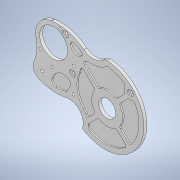
# Autodesk Inventor part: 足内フレーム
Saved by Autodesk Inventor 2022.2 (Build 262287010, 287A)
## iProperties
Created: 2022-01-10
Part Number: 足内フレーム
Material: Aluminum 2014-T4
Document SubType Name: Modeling
Designer: acps
Density: 2.8 g/cm^3
Appearance: Satin
Author: acps
Autodesk Inventor part; units mm, degrees
ref_plane "YZ Plane" through (0, 0, 0) normal (1, 0, 0) x (0, 1, 0)
ref_plane "XZ Plane" through (0, 0, 0) normal (0, 1, 0) x (-1, 0, 0)
ref_plane "XY Plane" through (0, 0, 0) normal (0, 0, 1) x (1, 0, 0)
sketch "Sketch2" plane through (0, 0, 0) normal (0, 0, 1) x (1, 0, 0)
  circle A0 centre (46.4683, 30) radius 14
  circle A1 centre (66.4734, 20) radius 20.5 construction
  circle A2 centre (100, 0) radius 30 construction
  circle A3 centre (123.045, 25) radius 1.25
  circle A4 centre (100, 0) radius 3 construction
  circle A5 centre (35, 0) radius 6.025 construction
  circle A6 centre (35, 0) radius 9
  arc A7 (26.7096, 3.5028) -> (28.866, 26.2368) centre (-8.2942, 18.2924) ccw
  arc A8 (44, 47.83) -> (28.866, 26.2368) centre (46.4683, 30) ccw
  arc A9 (110.6259, 39.2116) -> (45.1112, 47.9488) centre (57.174, -111.5959) ccw construction
  arc A10 (91.0837, -36) -> (110.6259, 39.2116) centre (97.597, 2.4523) ccw
  arc A11 (28.683, 27.2278) -> (91.0837, -36) centre (103.7763, 38.9326) ccw construction
  circle A12 centre (58.3063, 43.4) radius 1.5
  arc A13 (44.5539, 47.9057) -> (44, 47.83) centre (65.9403, -110.6586) ccw
  arc A14 (76.7854, 39.1678) -> (44.5539, 47.9057) centre (50.3015, 5.2915) ccw
  arc A15 (76.7854, 39.1678) -> (96.2775, 40.0369) centre (86.0239, 50.9851) ccw
  arc A16 (100.004, 41.3779) -> (96.2775, 40.0369) centre (99.6954, 36.3875) ccw
  arc A17 (91.0837, -36) -> (100.004, 41.3779) centre (97.597, 2.4523) ccw
  arc A18 (75.52, -28.3291) -> (58.8706, -11.0424) centre (62.0019, -24.6877) ccw
  arc A19 (31.2271, -8.171) -> (58.8706, -11.0424) centre (49.2531, 30.8683) ccw
  arc A20 (75.52, -28.3291) -> (76.4189, -30.5623) centre (77.4512, -28.8493) ccw
  arc A21 (76.4189, -30.5623) -> (91.0837, -36) centre (98.098, 5.4101) ccw
  circle A22 centre (58.3063, 43.4) radius 1.5
  circle A23 centre (123.045, 25) radius 1.25
  circle A24 centre (100, 0) radius 3 construction
  circle A25 centre (100, 0) radius 8.525
  circle A26 centre (65.359, 13) radius 1.25
  arc A27 (131.5793, 3.5511) -> (107.9544, 34.8363) centre (97.597, 2.4523) ccw construction
  circle A28 centre (66.4734, 20) radius 1.5
  circle A29 centre (66.299, -4.4994) radius 4 construction
  circle A30 centre (66.299, -4.4994) radius 1.5
  circle A31 centre (66.299, -4.4994) radius 3 construction
  circle A32 centre (53.0056, 45.2) radius 1.25
  arc A33 (59.6568, 44.1821) -> (46.2779, 45.0886) centre (50.3015, 5.2915) ccw construction
  circle A34 centre (45.1, 8.5) radius 1.25
  circle A35 centre (33, 18) radius 1.25
  arc A36 (31.0568, 25.3067) -> (30.8433, 25.9979) centre (-68.6067, -5.1096) ccw construction
  line L0 (51.7556, 0) -> (32.0278, 0) construction
  circle A37 centre (35, 0) radius 1.5
  point P0 (0, 0)
  point P1 (0, 0)
  point P2 (86.6921, 36)
  point P3 (61.5525, 46.7935)
  point P4 (110.6259, 39.2116)
  dimension "d0" = 12.05
  dimension "d1" = 18
  dimension "d4" = 4
  dimension "d6" = 15
  dimension "d7" = 14
  dimension "d8" = 2
  dimension "d9" = 43
  dimension "d10" = 5
  dimension "d11" = 43
  dimension "d12" = 36
  dimension "d13" = 44
  dimension "d14" = 42
  dimension "d15" = 74
  dimension "d16" = 118
  dimension "d18" = 110.6259
  dimension "d21" = 17.05
  dimension "d22" = 2.5
  dimension "d23" = 37
  dimension "d24" = 13
  dimension "d26" = 3
  dimension "d27" = 2.5
  dimension "d28" = 25
  dimension "d29" = 5
  dimension "d35" = 3
  dimension "d36" = 8
  dimension "d37" = 3
  dimension "d38" = 6
  dimension "d39" = 2.5
  dimension "d40" = 3
  dimension "d42" = 45.2
  dimension "d43" = 2.5
  dimension "d44" = 8.5
  dimension "d45" = 45.1
  dimension "d46" = 2.5
  dimension "d50" = 65.359
  dimension "d51" = 35
  dimension "d52" = 38
  dimension "d53" = 18
  dimension "d54" = 33
  dimension "d116" = 3
  constraints: 41 point on circle, 37 centre point, 16 tangent, 9 coincident, 6 concentric, 2 end point, 2 horizontal, 1 point on line, 14 other
  measures "d0" diameter of A5
  measures "d1" diameter of A6
  measures "d4" radial gap between concentric circles of A8 A0
  measures "d6" radius of A15
  measures "d7" radius of A18
  measures "d8" radius of A20
  measures "d9" radius of A19
  measures "d10" radius of A16
  measures "d11" radius of A14
  measures "d12" vertical distance of point (0, 0) point (86.692, 36)
  measures "d13" horizontal distance of point (0, 0) A8.start
  measures "d14" radius of A21
  measures "d18" horizontal distance of point (0, 0) A10.end
  measures "d21" diameter of A25
  measures "d22" diameter of A26
  measures "d23" distance of A2.centre A26.centre
  measures "d24" vertical distance of point (0, 0) A26.centre
  measures "d26" diameter of A12
  measures "d27" diameter of A3
  measures "d28" vertical distance of point (0, 0) A3.centre
  measures "d29" radial gap between concentric circles of A10 A27
  measures "d35" diameter of A28
  measures "d36" diameter of A29
  measures "d37" diameter of A30
  measures "d38" diameter of A31
  measures "d39" diameter of A32
  measures "d40" radial gap between concentric circles of A14 A33
  measures "d42" vertical distance of point (0, 0) A32.centre
  measures "d43" diameter of A34
  measures "d44" vertical distance of point (0, 0) A34.centre
  measures "d45" horizontal distance of point (0, 0) A34.centre
  measures "d46" diameter of A35
  measures "d50" horizontal distance of point (0, 0) A26.centre
  measures "d51" distance of A6.centre point (0, 0)
  measures "d52" radius of A7
  measures "d53" vertical distance of point (0, 0) A35.centre
  measures "d54" horizontal distance of point (0, 0) A35.centre
  measures "d116" diameter of A37
extrude "Extrusion1" add sketch "Sketch2" against normal blind 3
sketch "Sketch3" plane through (0, 0, 0) normal (0, 0, 1) x (1, 0, 0)
  circle A0 centre (58.3063, 43.4) radius 3
  circle A1 centre (65.359, 13) radius 3
  circle A2 centre (123.045, 25) radius 1.25 projected
  circle A3 centre (123.045, 25) radius 3
  point P0 (0, 0)
  dimension "d30" = 6
  dimension "d31" = 6
  dimension "d32" = 6
  constraints: 3 centre point, 3 coincident
  measures "d30" diameter of A0
  measures "d31" diameter of A1
  measures "d32" diameter of A3
extrude "Extrusion2" cut sketch "Sketch3" against normal blind 1 contours A0 | A1 | A2 | A3
sketch "Sketch4" plane through (0, 0, 0) normal (0, 0, 1) x (1, 0, 0)
  arc A0 (83.9638, 31.0915) -> (98.805, 35.6018) centre (86.0239, 50.9851) ccw
  arc A1 (76.7854, 39.1678) -> (96.2775, 40.0369) centre (86.0239, 50.9851) ccw projected
  circle A2 centre (66.4734, 20) radius 1.5 projected
  arc A3 (91.0837, -36) -> (100.004, 41.3779) centre (97.597, 2.4523) ccw projected
  circle A4 centre (100, 0) radius 8.525 projected
  arc A5 (72.3356, 17.192) -> (72.9578, 20.4509) centre (66.4734, 20) ccw
  circle A6 centre (46.4683, 30) radius 14 projected
  arc A7 (101.0246, 36.2791) -> (98.805, 35.6018) centre (100.7221, 33.2943) ccw
  arc A8 (115.5935, 31.2989) -> (101.0246, 36.2791) centre (97.597, 2.4523) ccw
  arc A9 (117.3038, 26.7431) -> (124.0841, 19.0907) centre (123.045, 25) ccw
  circle A10 centre (123.045, 25) radius 3 projected
  arc A11 (128.4007, 16.8443) -> (124.0841, 19.0907) centre (124.7768, 15.1511) ccw
  arc A12 (83.3223, -28.406) -> (128.4007, 16.8443) centre (97.597, 2.4523) ccw
  arc A13 (81.0017, -24.7603) -> (83.3223, -28.406) centre (85.0017, -24.7756) ccw
  arc A14 (81.0017, -24.7603) -> (76.328, -12.2073) centre (62.0019, -24.6877) ccw
  arc A15 (75.52, -28.3291) -> (58.8706, -11.0424) centre (62.0019, -24.6877) ccw projected
  circle A16 centre (66.299, -4.4994) radius 1.5 projected
  circle A17 centre (100, 0) radius 15.525
  arc A18 (48.6036, -7.1262) -> (57.9971, -6.112) centre (49.2531, 30.8683) ccw
  arc A19 (44.8283, -2.0195) -> (48.6036, -7.1262) centre (48.672, -3.1268) ccw
  arc A20 (31.2271, -8.171) -> (58.8706, -11.0424) centre (49.2531, 30.8683) ccw projected
  arc A21 (72.3356, 17.192) -> (76.328, -12.2073) centre (96.6862, 5.5281) ccw
  arc A22 (48.6524, 4.6231) -> (44.8283, -2.0195) centre (60.2031, -6.4485) ccw
  arc A23 (62.2417, 5.4118) -> (48.6524, 4.6231) centre (55.8716, -2.2967) ccw
  arc A24 (62.4749, -0.5464) -> (62.2417, 5.4118) centre (59.6936, 2.3284) ccw
  arc A25 (62.4749, -0.5464) -> (60.9598, -3.1794) centre (66.299, -4.4994) ccw
  arc A26 (54.145, 12.6119) -> (43.432, 4.4478) centre (60.2031, -6.4485) ccw construction
  circle A27 centre (45.1, 8.5) radius 1.25 projected
  arc A28 (67.6549, 6.9852) -> (54.9349, 12.674) centre (55.8716, -2.2967) ccw construction
  circle A29 centre (65.359, 13) radius 3 projected
  arc A30 (57.9971, -6.112) -> (60.9598, -3.1794) centre (57.0767, -2.2194) ccw
  arc A31 (43.9376, 3.3219) -> (41.8928, -7.3744) centre (48.672, -3.1268) ccw construction
  arc A32 (83.9638, 31.0915) -> (72.9578, 20.4509) centre (82.9337, 21.1447) ccw
  arc A33 (117.3038, 26.7431) -> (115.5935, 31.2989) centre (113.4763, 27.9051) ccw
  line L0 (122.5344, -20.6589) -> (111.8754, -10)
  line L1 (119.6469, -23.4283) -> (108.9231, -12.7045)
  line L2 (117.9886, 21.77) -> (108.9231, 12.7045)
  line L3 (121.1745, 19.299) -> (111.8754, 10)
  line L4 (0, 0) -> (194.5551, 0) construction
  line L5 (91.0769, 12.7045) -> (75.7157, 28.0657)
  line L6 (88.1246, 10) -> (73.5429, 24.5817)
  line L7 (88.1246, -10) -> (79.8771, -18.2475)
  line L8 (91.0769, -12.7045) -> (80.9144, -22.867)
  arc A34 (67.721, 40.1851) -> (63.3889, 37.7183) centre (66.381, 37.5009) ccw
  arc A35 (74.5126, 35.8664) -> (67.721, 40.1851) centre (50.3015, 5.2915) ccw
  arc A36 (74.7817, 32.9878) -> (74.5126, 35.8664) centre (73.271, 34.2984) ccw
  arc A37 (63.3889, 37.7183) -> (74.7817, 32.9878) centre (69.8718, 37.2473) ccw
  arc A38 (76.7854, 39.1678) -> (44.5539, 47.9057) centre (50.3015, 5.2915) ccw projected
  arc A39 (59.4664, 38.6529) -> (65.1004, 27.8941) centre (69.8718, 37.2473) ccw construction
  arc A40 (66.3457, 44.5008) -> (59.4046, 38.0749) centre (66.381, 37.5009) ccw construction
  circle A41 centre (58.3063, 43.4) radius 3 projected
  point P0 (85.9957, -17.7858)
  dimension "d56" = 5
  dimension "d64" = 5
  dimension "d65" = 3
  dimension "d66" = 3
  dimension "d67" = 5
  dimension "d68" = 4
  dimension "d69" = 5
  dimension "d72" = 4
  dimension "d73" = 7
  dimension "d75" = 5
  dimension "d76" = 4
  dimension "d79" = 5
  dimension "d82" = 27
  dimension "d83" = 4
  dimension "d84" = 5
  dimension "d85" = 4
  dimension "d86" = 4
  dimension "d87" = 4
  dimension "d88" = 16
  dimension "d89" = 10
  dimension "d90" = 4
  dimension "d91" = 10
  dimension "d92" = 4
  dimension "d94" = 4
  dimension "d95" = 4
  dimension "d96" = 10
  dimension "d97" = 45
  dimension "d99" = 10
  dimension "d100" = 45
  dimension "d101" = 135
  dimension "d102" = 10
  dimension "d103" = 4
  dimension "d104" = 45
  dimension "d105" = 4
  dimension "d106" = 10
  dimension "d109" = 4
  dimension "d110" = 4
  dimension "d111" = 4
  dimension "d112" = 2
  dimension "d113" = 6.5
  dimension "d114" = 3
  constraints: 64 point on circle, 28 centre point, 27 tangent, 18 end point, 14 concentric, 4 parallel, 1 coincident, 1 horizontal, 1 midpoint, 10 other
  measures "d56" radial gap between concentric circles of A1 A0
  measures "d64" radial gap between concentric circles of A3 A8
  measures "d65" radius of A7
  measures "d66" radial gap between concentric circles of A9 A10
  measures "d67" radial gap between concentric circles of A12 A3
  measures "d68" radius of A11
  measures "d69" radial gap between concentric circles of A15 A14
  measures "d72" radius of A13
  measures "d75" radial gap between concentric circles of A20 A18
  measures "d76" radius of A19
  measures "d79" radial gap between concentric circles of A2 A5
  measures "d82" radius of A21
  measures "d83" radial gap between concentric circles of A22 A26
  measures "d84" radial gap between concentric circles of A23 A28
  measures "d85" radius of A24
  measures "d86" radial gap between concentric circles of A16 A25
  measures "d87" radius of A30
  measures "d88" radius of A22
  measures "d89" radius of A23
  measures "d90" radial gap between concentric circles of A31 A19
  measures "d91" radius of A32
  measures "d92" radius of A33
  measures "d94" distance between parallel lines of L0 L1
  measures "d95" distance between parallel lines of L2 L3
  measures "d96" vertical distance of L4.start L3.end
  measures "d97" angle of L4 L0
  measures "d99" vertical distance of L4.start L0.end
  measures "d100" angle of L4 L3
  measures "d101" angle of L4 L6
  measures "d102" vertical distance of L4.start L6.start
  measures "d103" distance between parallel lines of L6 L5
  measures "d104" angle of L4 L7
  measures "d105" distance from line of point (85.996, -17.786) L7
  measures "d106" vertical distance of L4.start L7.start
  measures "d109" radial gap between concentric circles of A34 A40
  measures "d110" radial gap between concentric circles of A38 A35
  measures "d111" radial gap between concentric circles of A39 A37
  measures "d112" radius of A36
  measures "d113" radius of A37
  measures "d114" radius of A34
extrude "Extrusion3" cut sketch "Sketch4" against normal blind 1.3 contours A0 A7 A8 A33 A9 L2 A17 L5 A32 | L6 A17 L7 A14 A21 A5 A32 | L3 A9 A11 A12 L0 A17 | A17 L1 A12 A13 A14 L8 | A19 A22 A23 A24 A25 A30 A18 | A35 A36 A37 A34
fillet "Fillet1" radius 2 16 edges at (111.8754, 10, -0.65) (111.8754, -10, -0.65) (122.5344, -20.6589, -0.65) (108.9231, -12.7045, -0.65) (119.6469, -23.4283, -0.65) (91.0769, -12.7045, -0.65) (88.1246, -10, -0.65) (88.1246, 10, -0.65) (73.5429, 24.5817, -0.65) (79.8771, -18.2475, -0.65) (91.0769, 12.7045, -0.65) (75.7157, 28.0657, -0.65) (108.9231, 12.7045, -0.65) (117.9886, 21.77, -0.65) (80.9144, -22.867, -0.65) (121.1745, 19.299, -0.65)
sketch "export" plane through (0, 0, 0) normal (0, 0, 1) x (1, 0, 0)
  line L0 (113.1045, 11.2291) -> (120.3869, 18.5115) projected
  arc A0 (122.1121, 19.073) -> (120.3869, 18.5115) centre (121.8011, 17.0973) ccw projected
  arc A1 (122.1121, 19.073) -> (124.0841, 19.0907) centre (123.045, 25) ccw projected
  arc A2 (128.4007, 16.8443) -> (124.0841, 19.0907) centre (124.7768, 15.1511) ccw projected
  arc A3 (123.9839, -18.9891) -> (128.4007, 16.8443) centre (97.597, 2.4523) ccw projected
  arc A4 (121.0175, -19.1421) -> (123.9839, -18.9891) centre (122.4317, -17.7279) ccw projected
  line L1 (121.0175, -19.1421) -> (113.1045, -11.2291) projected
  arc A5 (112.8618, -8.6948) -> (113.1045, -11.2291) centre (114.5187, -9.8149) ccw projected
  arc A6 (112.8618, -8.6948) -> (112.8618, 8.6948) centre (100, 0) ccw projected
  arc A7 (113.1045, 11.2291) -> (112.8618, 8.6948) centre (114.5187, 9.8149) ccw projected
  arc A8 (48.6524, 4.6231) -> (44.8283, -2.0195) centre (60.2031, -6.4485) ccw projected
  arc A9 (62.2417, 5.4118) -> (48.6524, 4.6231) centre (55.8716, -2.2967) ccw projected
  arc A10 (62.4749, -0.5464) -> (62.2417, 5.4118) centre (59.6936, 2.3284) ccw projected
  arc A11 (62.4749, -0.5464) -> (60.9598, -3.1794) centre (66.299, -4.4994) ccw projected
  arc A12 (57.9971, -6.112) -> (60.9598, -3.1794) centre (57.0767, -2.2194) ccw projected
  arc A13 (48.6036, -7.1262) -> (57.9971, -6.112) centre (49.2531, 30.8683) ccw projected
  arc A14 (44.8283, -2.0195) -> (48.6036, -7.1262) centre (48.672, -3.1268) ccw projected
  line L2 (89.9475, 13.8339) -> (77.2718, 26.5097) projected
  arc A15 (77.6241, 29.6187) -> (77.2718, 26.5097) centre (78.686, 27.9239) ccw projected
  arc A16 (83.9638, 31.0915) -> (77.6241, 29.6187) centre (82.9337, 21.1447) ccw projected
  arc A17 (83.9638, 31.0915) -> (98.805, 35.6018) centre (86.0239, 50.9851) ccw projected
  arc A18 (101.0246, 36.2791) -> (98.805, 35.6018) centre (100.7221, 33.2943) ccw projected
  arc A19 (115.5935, 31.2989) -> (101.0246, 36.2791) centre (97.597, 2.4523) ccw projected
  arc A20 (117.3038, 26.7431) -> (115.5935, 31.2989) centre (113.4763, 27.9051) ccw projected
  arc A21 (117.3038, 26.7431) -> (117.4325, 22.8787) centre (123.045, 25) ccw projected
  arc A22 (116.9759, 20.7573) -> (117.4325, 22.8787) centre (115.5617, 22.1715) ccw projected
  line L3 (116.9759, 20.7573) -> (110.0525, 13.8339) projected
  arc A23 (107.6525, 13.508) -> (110.0525, 13.8339) centre (108.6383, 15.2481) ccw projected
  arc A24 (107.6525, 13.508) -> (92.3475, 13.508) centre (100, 0) ccw projected
  arc A25 (89.9475, 13.8339) -> (92.3475, 13.508) centre (91.3617, 15.2481) ccw projected
  line L4 (110.0525, -13.8339) -> (118.0628, -21.8442) projected
  arc A26 (117.8393, -24.8653) -> (118.0628, -21.8442) centre (116.6485, -23.2584) ccw projected
  arc A27 (83.3223, -28.406) -> (117.8393, -24.8653) centre (97.597, 2.4523) ccw projected
  arc A28 (81.0017, -24.7603) -> (83.3223, -28.406) centre (85.0017, -24.7756) ccw projected
  arc A29 (81.0017, -24.7603) -> (80.978, -23.7347) centre (62.0019, -24.6877) ccw projected
  arc A30 (81.5612, -22.2202) -> (80.978, -23.7347) centre (82.9754, -23.6344) ccw projected
  line L5 (81.5612, -22.2202) -> (89.9475, -13.8339) projected
  arc A31 (92.3475, -13.508) -> (89.9475, -13.8339) centre (91.3617, -15.2481) ccw projected
  arc A32 (92.3475, -13.508) -> (107.6525, -13.508) centre (100, 0) ccw projected
  arc A33 (110.0525, -13.8339) -> (107.6525, -13.508) centre (108.6383, -15.2481) ccw projected
  line L6 (86.8955, -11.2291) -> (81.9314, -16.1932) projected
  arc A34 (78.7538, -15.7227) -> (81.9314, -16.1932) centre (80.5172, -14.779) ccw projected
  arc A35 (78.7538, -15.7227) -> (76.328, -12.2073) centre (62.0019, -24.6877) ccw projected
  arc A36 (72.3356, 17.192) -> (76.328, -12.2073) centre (96.6862, 5.5281) ccw projected
  arc A37 (72.3356, 17.192) -> (72.9685, 20.2517) centre (66.4734, 20) ccw projected
  arc A38 (76.3813, 21.7433) -> (72.9685, 20.2517) centre (74.967, 20.3291) ccw projected
  line L7 (76.3813, 21.7433) -> (86.8955, 11.2291) projected
  arc A39 (87.1382, 8.6948) -> (86.8955, 11.2291) centre (85.4813, 9.8149) ccw projected
  arc A40 (87.1382, 8.6948) -> (87.1382, -8.6948) centre (100, 0) ccw projected
  arc A41 (86.8955, -11.2291) -> (87.1382, -8.6948) centre (85.4813, -9.8149) ccw projected
  arc A42 (74.7817, 32.9878) -> (74.5126, 35.8664) centre (73.271, 34.2984) ccw projected
  arc A43 (63.3889, 37.7183) -> (74.7817, 32.9878) centre (69.8718, 37.2473) ccw projected
  arc A44 (67.721, 40.1851) -> (63.3889, 37.7183) centre (66.381, 37.5009) ccw projected
  arc A45 (74.5126, 35.8664) -> (67.721, 40.1851) centre (50.3015, 5.2915) ccw projected
  circle A46 centre (123.045, 25) radius 3 projected
  circle A47 centre (65.359, 13) radius 3 projected
  circle A48 centre (58.3063, 43.4) radius 3 projected
  arc A49 (26.7096, 3.5028) -> (28.866, 26.2368) centre (-8.2942, 18.2924) ccw projected
  arc A50 (26.7096, 3.5028) -> (31.2271, -8.171) centre (35, 0) ccw projected
  arc A51 (31.2271, -8.171) -> (58.8706, -11.0424) centre (49.2531, 30.8683) ccw projected
  arc A52 (75.52, -28.3291) -> (58.8706, -11.0424) centre (62.0019, -24.6877) ccw projected
  arc A53 (75.52, -28.3291) -> (76.4189, -30.5623) centre (77.4512, -28.8493) ccw projected
  arc A54 (76.4189, -30.5623) -> (91.0837, -36) centre (98.098, 5.4101) ccw projected
  arc A55 (91.0837, -36) -> (100.004, 41.3779) centre (97.597, 2.4523) ccw projected
  arc A56 (100.004, 41.3779) -> (96.2775, 40.0369) centre (99.6954, 36.3875) ccw projected
  arc A57 (76.7854, 39.1678) -> (96.2775, 40.0369) centre (86.0239, 50.9851) ccw projected
  arc A58 (76.7854, 39.1678) -> (44.5539, 47.9057) centre (50.3015, 5.2915) ccw projected
  arc A59 (44.5539, 47.9057) -> (44, 47.83) centre (65.9403, -110.6586) ccw projected
  arc A60 (44, 47.83) -> (28.866, 26.2368) centre (46.4683, 30) ccw projected
  circle A61 centre (33, 18) radius 1.25 projected
  circle A62 centre (45.1, 8.5) radius 1.25 projected
  circle A63 centre (66.4734, 20) radius 1.5 projected
  circle A64 centre (53.0056, 45.2) radius 1.25 projected
  circle A65 centre (66.299, -4.4994) radius 1.5 projected
  circle A66 centre (100, 0) radius 8.525 projected
  circle A67 centre (46.4683, 30) radius 14 projected
  circle A68 centre (65.359, 13) radius 1.25 projected
  circle A69 centre (58.3063, 43.4) radius 1.5 projected
  circle A70 centre (123.045, 25) radius 1.25 projected
  point P0 (0, 0)
sketch "Sketch6" plane through (0, 0, -3) normal (0, 0, -1) x (-1, 0, 0)
  circle A0 centre (-66.4734, 20) radius 1.5 projected
  circle A1 centre (-66.4734, 20) radius 4.5
  point P0 (0, 0)
  dimension "d117" = 3
  constraints: 1 centre point
  measures "d117" radial gap between concentric circles of A0 A1
extrude "Extrusion4" cut sketch "Sketch6" against normal blind 1
body "Solid1"
